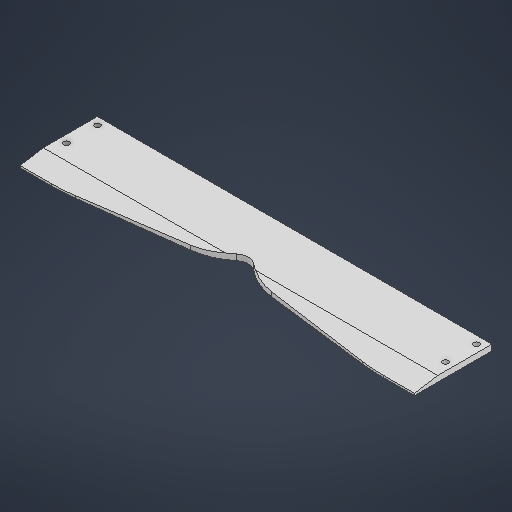
# Autodesk Inventor part: lady brown aligner
Saved by Autodesk Inventor 2025 (Build 290162000, 162)
## iProperties
Created: 2025-02-05
Part Number: lady brown aligner
Material: Generic
Document SubType Name: Modeling
Designer: Juan
Density: 1 g/cm^3
Appearance: Default
Author: Juan
Autodesk Inventor part; units mm, degrees
ref_plane "YZ Plane" through (0, 0, 0) normal (1, 0, 0) x (0, 1, 0)
ref_plane "XZ Plane" through (0, 0, 0) normal (0, 1, 0) x (-1, 0, 0)
ref_plane "XY Plane" through (0, 0, 0) normal (0, 0, 1) x (1, 0, 0)
sketch "Sketch1" plane through (0, 0, 0) normal (0, 1, 0) x (-1, 0, 0)
  line L0 (0, 0) -> (-323.85, 0)
  line L1 (-323.85, 0) -> (-323.85, 63.5)
  line L2 (-323.85, 63.5) -> (0, 63.5)
  line L3 (0, 63.5) -> (0, 0)
  line L4 (-323.85, 0) -> (-323.85, 6.35)
  line L5 (0, 0) -> (-6.35, 0)
  line L6 (-323.85, 0) -> (-317.5, 0)
  line L7 (-323.85, 6.35) -> (-317.5, 6.35)
  line L8 (-317.5, 6.35) -> (-317.5, 31.75)
  line L9 (-6.35, 0) -> (-6.35, 6.35)
  line L10 (-6.35, 6.35) -> (-6.35, 31.75)
  circle A0 centre (-6.35, 6.35) radius 2.3241
  circle A1 centre (-6.35, 31.75) radius 2.3241
  circle A2 centre (-317.5, 31.75) radius 2.3241
  circle A3 centre (-317.5, 6.35) radius 2.3241
  line L11 (-161.925, 0) -> (-161.925, 38.1)
  line L12 (-161.925, 63.5) -> (-288.925, 63.5)
  line L13 (-161.925, 63.5) -> (-34.925, 63.5)
  line L14 (-161.925, 63.5) -> (-161.925, 38.1)
  line L15 (-161.925, 63.5) -> (-161.925, 57.15)
  circle A4 centre (-161.925, 63.5) radius 9.525
  circle A5 centre (-161.925, 49.2261) radius 11.1261
  line L16 (-288.925, 63.5) -> (-171.45, 43.4759)
  line L17 (-34.925, 63.5) -> (-152.4, 43.4759)
  line L18 (-288.925, 63.5) -> (-173.0511, 49.2261)
  line L19 (-34.925, 63.5) -> (-150.7989, 49.2261)
  dimension "d0" = 323.85
  dimension "d1" = 63.5
  dimension "d2" = 6.35
  dimension "d3" = 6.35
  dimension "d4" = 6.35
  dimension "d5" = 25.4
  dimension "d6" = 6.35
  dimension "d7" = 25.4
  dimension "d8" = 4.6482
  dimension "d9" = 4.6482
  dimension "d10" = 4.6482
  dimension "d11" = 4.6482
  dimension "d12" = 38.1
  dimension "d13" = 127
  dimension "d14" = 127
  dimension "d15" = 6.35
  dimension "d16" = 19.05
  constraints: 40 end point, 8 point on line, 6 centre point, 5 coincident, 5 perpendicular, 4 point on circle, 2 horizontal, 2 midpoint, 2 vertical, 1 symmetric about line
  measures "d0" distance of L0.start L0.end
  measures "d1" distance of L0.end L1.end
  measures "d2" distance of L0.end L4.end
  measures "d3" distance of L0.start L5.end
  measures "d4" distance of L0.end L6.end
  measures "d5" distance of L7.end L8.end
  measures "d6" distance of L5.end L9.end
  measures "d7" distance of L9.end L10.end
  measures "d8" diameter of A0
  measures "d9" diameter of A1
  measures "d10" diameter of A2
  measures "d11" diameter of A3
  measures "d12" distance of L11.start L11.end
  measures "d13" distance of L12.start L12.end
  measures "d14" distance of L12.start L13.end
  measures "d15" distance of L12.start L15.end
  measures "d16" diameter of A4
extrude "Extrusion1" add sketch "Sketch1" along normal blind 4.7625 contours L0 L11 A5 L17 L2 L3 | L0 L1 L2 L16 A5 L11
extrude "Extrusion2" add sketch "Sketch1" along normal blind 4.7625 contours L17 A5 L19 | L16 L18 A5
fillet "Fillet1" radius 50.8 2 edges at (173.0511, 2.3813, 49.2261) (150.7989, 2.3813, 49.2261)
fillet "Fillet2" radius 152.4 2 edges at (288.925, 2.3813, 63.5) (34.925, 2.3813, 63.5)
sketch "Sketch2" plane through (0, 0, 0) normal (-1, 0, 0) x (0, 0, 1)
  line L0 (63.5, 0) -> (63.5, 4.7625) projected
  line L1 (63.5, 0) -> (63.5, 1.5875)
  line L2 (63.5, 1.5875) -> (50.4087, 4.7625)
  line L3 (0, 4.7625) -> (63.5, 4.7625) projected
  line L4 (63.5, 4.7625) -> (50.4087, 4.7625)
  line L5 (63.5, 1.5875) -> (63.5, 4.7625)
  line L6 (63.5, 1.5875) -> (44.4761, 4.7625)
  line L7 (44.4761, 4.7625) -> (50.4087, 4.7625)
  point P0 (0, 0)
  dimension "d24" = 1.5875
  constraints: 12 end point, 3 point on line, 2 collinear, 1 perpendicular
  measures "d24" distance of L0.start L1.end
extrude "Extrusion3" cut sketch "Sketch2" against normal through all
body "Solid1"
